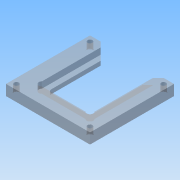
# Autodesk Inventor part: Tunel_OdourPortSlidingMechanism
Saved by Autodesk Inventor 2016 (Build 200138000, 138)
## iProperties
Created: 2015-01-22
Part Number: Tunel_OdourPortSlidingMechanism
Material: Polycarbonat, klar
Document SubType Name: Modeling
Designer: Gero Hofmann
Density: 1.2 g/cm^3
Appearance: Polycarbonat - klar
Author: Gero Hofmann
Autodesk Inventor part; units mm, degrees
ref_plane "YZ Plane" through (0, 0, 0) normal (1, 0, 0) x (0, 1, 0)
ref_plane "XZ Plane" through (0, 0, 0) normal (0, 1, 0) x (-1, 0, 0)
ref_plane "XY Plane" through (0, 0, 0) normal (0, 0, 1) x (1, 0, 0)
sketch "Skizze1" plane through (0, 0, 0) normal (0, 0, 1) x (1, 0, 0)
  line L0 (40, 40) -> (40, -40)
  line L1 (40, -40) -> (-40, -40)
  line L2 (-40, -40) -> (-40, 40)
  line L3 (-40, 40) -> (40, -40) construction
  line L4 (40, 40) -> (-40, -40) construction
  line L5 (-20, 40) -> (-20, -20)
  line L6 (-20, -20) -> (20, -20)
  line L7 (20, -20) -> (20, 40)
  line L8 (-40, 40) -> (-20, 40)
  line L9 (20, 40) -> (40, 40)
  point P0 (0, 0)
  dimension "d0" = 40
  dimension "d1" = 80
  constraints: 20 end point, 4 parallel, 2 equal length, 2 horizontal, 2 midpoint, 2 perpendicular, 2 other
  measures "d0" distance of L5.end L6.end
  measures "d1" distance of L0.end L1.end
extrude "Extrusion1" add sketch "Skizze1" along normal blind 10
sketch "Skizze2" plane through (0, 0, 10) normal (0, 0, 1) x (1, 0, 0)
  line L0 (-40, 40) -> (-40, -40) projected
  line L1 (40, 40) -> (20, 40) projected
  line L2 (20, 40) -> (20, -20) projected
  line L3 (20, -20) -> (-20, -20) projected
  line L4 (-20, -20) -> (-20, 40) projected
  line L5 (-20, 40) -> (-40, 40) projected
  line L6 (-25, 40) -> (-25, -20.7574)
  line L7 (-20.7574, -25) -> (20.7574, -25)
  line L8 (25, -20.7574) -> (25, 40)
  arc A0 (20.7574, -25) -> (25, -20.7574) centre (22.8787, -22.8787) ccw
  arc A1 (-25, -20.7574) -> (-20.7574, -25) centre (-22.8787, -22.8787) ccw
  line L9 (0, 56) -> (0, -56) construction
  point P0 (0, 0)
  dimension "d5" = 6
  dimension "d7" = 2.1213
  dimension "d8" = 2.1213
  dimension "d9" = 50
  dimension "d11" = 5
  dimension "d12" = 5
  constraints: 6 end point, 4 point on circle, 2 centre point, 2 point on line, 2 vertical, 1 equal radius, 1 horizontal, 1 horizontal alignment, 1 parallel, 2 other
  measures "d5" diameter of A0
  measures "d7" distance from line of L7 A0.centre
  measures "d8" distance from line of A0.centre L8
  measures "d9" distance between parallel lines of L8 L6
  measures "d11" distance between parallel lines of L6 L4
  measures "d12" distance between parallel lines of L7 L3
extrude "Extrusion2" cut sketch "Skizze2" against normal blind 6
fillet "Rundung1" radius 3 2 edges at (20, -20, 2) (-20, -20, 2)
chamfer "Fase1" distance 10 angle 45 2 edges at (-20, 40, 2) (20, 40, 2)
sketch "Skizze3" plane through (0, 0, 0) normal (0, 0, -1) x (-1, 0, 0)
  line L0 (-40, 40) -> (-20, 40) projected
  line L1 (-40, -40) -> (-40, 40) projected
  line L2 (40, -40) -> (-40, -40) projected
  line L3 (40, 40) -> (40, -40) projected
  line L4 (35, -35) -> (-35, -35)
  line L5 (-35, -35) -> (-35, 35)
  line L6 (-35, 35) -> (35, 35)
  line L7 (35, 35) -> (35, -35)
  line L8 (35, -35) -> (-35, 35) construction
  line L9 (-35, -35) -> (35, 35) construction
  point P0 (-21, 40)
  point P1 (0, 0)
  point P2 (0, 0)
  dimension "d22" = 5
  dimension "d23" = 5
  dimension "d24" = 5
  dimension "d25" = 5
  dimension "d33" = 70
  dimension "d34" = 70
  constraints: 12 end point, 2 midpoint, 2 parallel, 1 horizontal, 1 perpendicular
  measures "d22" distance between parallel lines of L3 L7
  measures "d23" distance between parallel lines of L2 L4
  measures "d24" distance between parallel lines of L1 L5
  measures "d25" distance between parallel lines of L0 L6
  measures "d33" distance of L5.end L6.end
  measures "d34" distance of L4.end L5.end
hole "Bohrung1" at (-35, 35, 0) at (-35, -35, 0) at (35, -35, 0) at (35, 35, 0) direction (0, 0, 1) diameter 4.5 end through all countersink diameter 10 countersink angle 90 clearance for "Innensechskant-Senkkopfschraube DIN EN ISO 10642" size "M4" standard "DIN"
equation "\"d8\" = d7"
equation "\"d12\" = d11"
equation "\"d23\" = d22"
equation "\"d24\" = d22"
equation "\"d25\" = d22"
